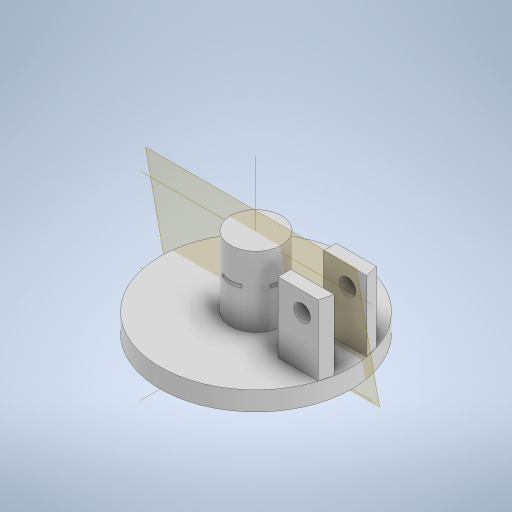
# Autodesk Inventor part: exp_latch_base_rev0
Saved by Autodesk Inventor 2024 (Build 280153000, 153)
## iProperties
Created: 2024-04-11
Part Number: exp_latch_base_rev0
Material: 一般
Document SubType Name: Modeling
Designer: Akio
Density: 1 g/cm^3
Appearance: 既定
Author: Akio
Autodesk Inventor part; units mm, degrees
ref_plane "XZ Plane" through (0, 0, 0) normal (0, 1, 0) x (-1, 0, 0)
ref_plane "XY Plane" through (0, 0, 0) normal (0, 0, 1) x (1, 0, 0)
sketch "スケッチ1" plane through (0, 0, 0) normal (0, 1, 0) x (-1, 0, 0)
  circle A0 centre (0, 0) radius 15
  dimension "d0" = 30
  constraints: 1 centre point, 1 coincident
  measures "d0" diameter of A0
extrude "押し出し1" add sketch "スケッチ1" along normal blind 3
sketch "スケッチ2" plane through (0, 3, 0) normal (0, 1, 0) x (1, 0, 0)
  circle A0 centre (0, 0) radius 15 projected
  line L0 (14.7817, -2.55) -> (8, -2.55)
  line L1 (8, -2.55) -> (8, -4.55)
  line L2 (8, 4.55) -> (8, 2.55)
  line L3 (-21, 0) -> (21, 0) projected
  line L4 (0, 21) -> (0, -21) projected
  line L5 (8, -4.55) -> (14.2933, -4.55)
  line L6 (14.7817, -2.55) -> (14.2933, -4.55)
  line L7 (8, 2.55) -> (14.7817, 2.55)
  line L8 (8, 2.55) -> (14.7817, 2.55) construction
  line L9 (8, 4.55) -> (14.2933, 4.55)
  line L10 (14.7817, 2.55) -> (14.2933, 4.55)
  point P0 (11.3908, -2.55)
  point P1 (8, -3.55)
  point P2 (8, 3.55)
  dimension "d16" = 2
  dimension "d27" = 8
  dimension "d28" = 2.55
  dimension "d29" = 8
  dimension "d31" = 2
  dimension "d33" = 2.55
  constraints: 18 end point, 4 horizontal, 4 point on circle, 3 midpoint, 1 collinear, 1 vertical
  measures "d16" distance of L0.end L1.end
  measures "d27" distance from line of L4 point (8, -3.55)
  measures "d28" distance between parallel lines of L3 L0
  measures "d29" distance from line of L4 point (8, 3.55)
  measures "d31" distance of L2.end L2.start
  measures "d33" distance between parallel lines of L3 L7
extrude "押し出し2" add sketch "スケッチ2" along normal blind 11 contours L7 L2 L9 L10 | L6 L5 L1 L0
sketch "スケッチ4" plane through (14.2933, 3, -4.55) normal (0, 0, -1) x (-1, 0, 0)
  circle A0 centre (2.5, 8) radius 1.3
  line L0 (29.2933, 0) -> (0, 0) projected
  line L1 (6.2933, 0) -> (6.2933, 11) projected
  line L2 (0, 0) -> (0, 11) projected
  point P0 (14.2933, -3)
  dimension "d34" = 2.6
  dimension "d35" = 8
  dimension "d42" = 2.5
  constraints: 1 centre point
  measures "d34" diameter of A0
  measures "d35" distance from line of L0 A0.centre
  measures "d42" distance from line of A0.centre L2
extrude "押し出し4" cut sketch "スケッチ4" against normal through all
sketch "スケッチ5" plane through (0, 3, 0) normal (0, 1, 0) x (1, 0, 0)
  circle A0 centre (0, 0) radius 4
  dimension "d39" = 8
  constraints: 1 centre point, 1 coincident
  measures "d39" diameter of A0
extrude "押し出し5" add sketch "スケッチ5" along normal blind 11
sketch "スケッチ6" plane through (0, 0, 0) normal (1, 0, 0) x (0, 1, 0)
  line L0 (3, -4.55) -> (3, 4.55) projected
  line L1 (3, -2.55) -> (3, -4.55) projected
  line L2 (3, 2.55) -> (3, -2.55) projected
  line L3 (3, 4.55) -> (3, 2.55) projected
  line L4 (0, -15) -> (0, 15) projected
  line L5 (0, -15) -> (3, -15) projected
  point P0 (0, 0)
  point P1 (13, 0)
  dimension "d43" = 15
  dimension "d44" = 10
  measures "d43" distance from line of L5 point (13, 0)
  measures "d44" distance from line of L0 point (13, 0)
ref_plane "作業平面1" through (0, 13, 0) normal (0, -0.1736, 0.9848) x (1, 0, 0)
sketch "スケッチ7" plane through (0, 13, 0) normal (0, -0.1736, 0.9848) x (1, 0, 0)
  line L0 (1.5, -3) -> (-1.5, -3)
  line L1 (1.5, -3) -> (1.5, -3.5)
  line L2 (1.5, -3.5) -> (-1.5, -3.5)
  line L3 (-1.5, -3.5) -> (-1.5, -3)
  line L4 (0, -19.2066) -> (0, 7.3889) projected
  line L5 (-21, 0) -> (21, 0) projected
  point P0 (0, -12.8025)
  point P1 (1.5, -3.25)
  dimension "d46" = 3
  dimension "d47" = 0.5
  dimension "d48" = 1.5
  dimension "d49" = 3
  constraints: 8 end point, 2 perpendicular, 1 horizontal, 1 midpoint, 1 vertical
  measures "d46" distance of L0.start L0.end
  measures "d47" distance of L0.start L1.end
  measures "d48" distance from line of L4 point (1.5, -3.25)
  measures "d49" distance between parallel lines of L0 L5
extrude "押し出し6" cut sketch "スケッチ7" along normal blind 10
pattern_circular "円形状パターン1" count 4 over 360 about axis through (0, 3, 0) along (0, 1, 0) of "押し出し6"
